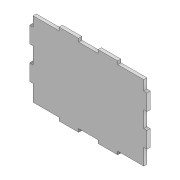
# Autodesk Inventor part: Lat 3
Saved by Autodesk Inventor 2022 (Build 260153000, 153)
## iProperties
Created: 2022-06-21
Part Number: Lat 3
Material: Generic
Document SubType Name: Modeling
Designer: ADMIN
Density: 1 g/cm^3
Appearance: Default
Author: ADMIN
Autodesk Inventor part; units mm, degrees
ref_plane "YZ Plane" through (0, 0, 0) normal (1, 0, 0) x (0, 1, 0)
ref_plane "XZ Plane" through (0, 0, 0) normal (0, 1, 0) x (-1, 0, 0)
ref_plane "XY Plane" through (0, 0, 0) normal (0, 0, 1) x (1, 0, 0)
sketch "Sketch1" plane through (0, 0, 0) normal (0, 0, 1) x (1, 0, 0)
  line L0 (-56.8722, -2.2872) -> (113.1278, -2.2872)
  line L1 (113.1278, -2.2872) -> (113.1278, 112.7128)
  line L2 (113.1278, 112.7128) -> (-56.8722, 112.7128)
  line L3 (-56.8722, 112.7128) -> (-56.8722, -2.2872)
  line L4 (-16.8722, 112.7128) -> (13.1278, 112.7128)
  line L5 (13.1278, 112.7128) -> (13.1278, 117.7128)
  line L6 (13.1278, 117.7128) -> (-16.8722, 117.7128)
  line L7 (-16.8722, 117.7128) -> (-16.8722, 112.7128)
  line L8 (43.1278, 112.7128) -> (73.1278, 112.7128)
  line L9 (73.1278, 112.7128) -> (73.1278, 117.7128)
  line L10 (73.1278, 117.7128) -> (43.1278, 117.7128)
  line L11 (43.1278, 117.7128) -> (43.1278, 112.7128)
  line L12 (-56.8722, 97.7128) -> (-61.8722, 97.7128)
  line L13 (-61.8722, 97.7128) -> (-61.8722, 72.7128)
  line L14 (-61.8722, 72.7128) -> (-56.8722, 72.7128)
  line L15 (-56.8722, 72.7128) -> (-56.8722, 97.7128)
  line L16 (-56.8722, 47.7128) -> (-61.8722, 47.7128)
  line L17 (-61.8722, 47.7128) -> (-61.8722, 22.7128)
  line L18 (-61.8722, 22.7128) -> (-56.8722, 22.7128)
  line L19 (-56.8722, 22.7128) -> (-56.8722, 47.7128)
  line L20 (28.1278, 112.7128) -> (28.1278, 0) construction
  line L21 (113.1278, 55.2128) -> (-59.3722, 55.2128) construction
  line L22 (13.1278, -2.2872) -> (13.1278, -7.2872)
  line L23 (13.1278, -7.2872) -> (-16.8722, -7.2872)
  line L24 (-16.8722, -7.2872) -> (-16.8722, -2.2872)
  line L25 (73.1278, -2.2872) -> (73.1278, -7.2872)
  line L26 (73.1278, -7.2872) -> (43.1278, -7.2872)
  line L27 (43.1278, -7.2872) -> (43.1278, -2.2872)
  line L28 (113.1278, 97.7128) -> (118.1278, 97.7128)
  line L29 (118.1278, 97.7128) -> (118.1278, 72.7128)
  line L30 (118.1278, 72.7128) -> (113.1278, 72.7128)
  line L31 (113.1278, 47.7128) -> (118.1278, 47.7128)
  line L32 (118.1278, 47.7128) -> (118.1278, 22.7128)
  line L33 (118.1278, 22.7128) -> (113.1278, 22.7128)
  line L34 (-56.8722, 55.2128) -> (115.6278, 55.2128) construction
  point P0 (0, 0)
  dimension "d0" = 170
  dimension "d1" = 115
  dimension "d2" = 30
  dimension "d3" = 5
  dimension "d4" = 30
  dimension "d5" = 5
  dimension "d6" = 30
  dimension "d7" = 40
  dimension "d8" = 5
  dimension "d9" = 25
  dimension "d10" = 5
  dimension "d11" = 25
  dimension "d12" = 25
  dimension "d13" = 15
  constraints: 70 end point, 18 symmetric about line, 10 parallel, 7 perpendicular, 5 horizontal, 4 point on line, 2 midpoint
  measures "d0" distance of L2.end L1.end
  measures "d1" distance of L1.end L0.end
  measures "d2" distance of L6.end L5.end
  measures "d3" distance of L5.end L4.end
  measures "d4" distance of L10.end L9.end
  measures "d5" distance of L9.end L8.end
  measures "d6" distance between parallel lines of L5 L11
  measures "d7" distance between parallel lines of L3 L7
  measures "d8" distance of L14.end L13.end
  measures "d9" distance of L13.end L12.end
  measures "d10" distance of L18.end L17.end
  measures "d11" distance of L17.end L16.end
  measures "d12" distance between parallel lines of L16 L14
  measures "d13" distance between parallel lines of L12 L2
extrude "Extrusion1" add sketch "Sketch1" along normal blind 5
body "Solid1"
